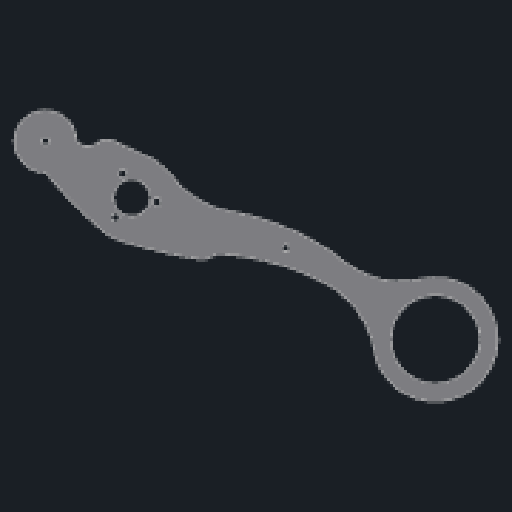
# Autodesk Inventor part: LowerLeg
Saved by Autodesk Inventor 2025.2 (Build 292293000, 293)
## iProperties
Created: 2020-05-17
Part Number: LowerLeg
Material: Generic
Document SubType Name: Sheet Metal
Designer: valer
Density: 1 g/cm^3
Sheet Metal Rule: Default
Appearance: Default
Author: valer
Autodesk Inventor part; units mm, degrees
ref_plane "YZ Plane" through (0, 0, 0) normal (1, 0, 0) x (0, 1, 0)
ref_plane "XZ Plane" through (0, 0, 0) normal (0, 1, 0) x (-1, 0, 0)
ref_plane "XY Plane" through (0, 0, 0) normal (0, 0, 1) x (1, 0, 0)
sketch "Base" plane through (0, 0, 0) normal (0, 0, 1) x (1, 0, 0)
  circle A0 centre (0, 0) radius 25.4
  arc A1 (296.4611, -175.8738) -> (140.4514, -91.7589) centre (131.6761, -294.7694) ccw
  arc A2 (110.2711, -36.5273) -> (55.3611, 0.3584) centre (-26.1088, -180.2356) ccw
  arc A3 (110.2711, -36.5273) -> (151.7939, -57.2356) centre (164.9104, 21.0482) ccw
  arc A4 (244.1, -98.1325) -> (151.7939, -57.2356) centre (118.2154, -257.642) ccw
  arc A5 (244.1, -98.1325) -> (322.9398, -136.302) centre (369.9847, 61.3771) ccw
  arc A6 (339.7063, -172.5127) -> (322.9398, -136.302) centre (317.0592, -161.0119) ccw
  arc A7 (296.4611, -175.8738) -> (339.7063, -172.5127) centre (317.0592, -161.0119) ccw
  line L0 (128.6011, -96.3262) -> (140.4514, -91.7589)
  line L1 (0, 0) -> (317.0592, -161.0119) construction
  circle A8 centre (317.0592, -161.0119) radius 25.4 construction
  arc A9 (0, -25.4) -> (128.6011, -96.3262) centre (153.166, 100.265) ccw
  line L2 (0, 0) -> (0, -25.4) construction
  arc A10 (55.3611, 0.3584) -> (42.3326, -1.2004) centre (50.1387, -11.2181) ccw
  arc A11 (25.4, -0.0141) -> (42.3326, -1.2004) centre (34.5266, 8.8174) ccw
  line L3 (110.2711, -36.5273) -> (102.4101, -52.0068) construction
  line L4 (50.1387, -11.2181) -> (44.3883, -22.5417) construction
  line L5 (140.4514, -91.7589) -> (148.7008, -75.5146) construction
  line L6 (244.1, -98.1325) -> (233.6726, -118.6658) construction
  line L7 (339.7063, -172.5127) -> (317.0592, -161.0119) construction
  dimension "d101" = 50.8
  dimension "d98" = 355.6
  dimension "d99" = 203.2
  dimension "d100" = 79.375
  dimension "d102" = 198.12
  dimension "d103" = 50.8
  dimension "d104" = 12.7
  dimension "d105" = 203.2
  dimension "d106" = 48
  dimension "d107" = 12.7
  dimension "d108" = 12.7
  dimension "d109" = 23.495
  dimension "d111" = 158.75
  dimension "d112" = 222.25
  dimension "d113" = 49.784
  dimension "d114" = 65.0748
  dimension "d115" = 51.9176
  dimension "d116" = 95.3008
  dimension "d117" = 93.5228
  measures "d98" distance of L1.start L1.end
  measures "d99" radius of A4
  measures "d100" radius of A3
  measures "d102" radius of A2
  measures "d103" diameter of A0
  measures "d104" radius of A10
  measures "d105" radius of A5
  measures "d106" angle of L1 L0
  measures "d107" distance of L0.start L0.end
  measures "d108" distance from line of L1 L4.start
  measures "d109" distance from line of L1 A11.centre
  measures "d111" distance from line of L1 A9.centre
  measures "d112" distance from line of L1 A5.centre
  measures "d113" distance from line of point (0, 0) L4
  measures "d114" distance from line of L4.end L3
  measures "d115" distance between parallel lines of L5 L3
  measures "d116" distance between parallel lines of L6 L5
  measures "d117" distance from line of A6.centre L6
extrude "Plate1" add sketch "Base" along normal blind 5
sketch "MountHoles" plane through (0, 0, 5) normal (0, 0, 1) x (1, 0, 0)
  arc A0 (296.4611, -175.8738) -> (322.9398, -136.302) centre (317.0592, -161.0119) ccw projected
  circle A1 centre (317.0592, -161.0119) radius 3.175
  circle A2 centre (0, 0) radius 3.175
  circle A3 centre (0, 0) radius 15.875 construction
  circle A4 centre (0, 15.875) radius 3.175
  line L0 (0, 15.875) -> (0, 0) construction
  circle A5 centre (-13.7482, 7.9375) radius 3.175
  circle A6 centre (-13.7482, -7.9375) radius 3.175
  circle A7 centre (0, -15.875) radius 3.175
  circle A8 centre (13.7482, -7.9375) radius 3.175
  circle A9 centre (13.7482, 7.9375) radius 3.175
  point P0 (278.6053, -195.7416)
  point P1 (14.9365, 6.9557)
  dimension "d40" = 31.75
  dimension "d38" = 6.35
  dimension "d39" = 6.35
  dimension "d43" = 360
  constraints: 8 centre point, 3 coincident, 2 end point, 1 equal radius, 1 vertical, 1 vertical alignment, 15 other
  measures "d38" diameter of A1
  measures "d39" diameter of A2
hole "MountHolesFeature" at (0, 0, 5) direction (0, 0, -1) diameter 6.35 end through all
fillet "SmallFilletsFeature" radius 8 2 edges at (140.4514, -91.7589, 2.5) (128.6011, -96.3262, 2.5)
sketch "WheelMountHole" plane through (0, 0, 5) normal (0, 0, 1) x (1, 0, 0)
  arc A0 (296.4611, -175.8738) -> (322.9398, -136.302) centre (317.0592, -161.0119) ccw projected
  circle A1 centre (317.0592, -161.0119) radius 6.35
  point P0 (0, 0)
  point P1 (278.6053, -195.7416)
  dimension "d83" = 12.7
  constraints: 1 centre point, 1 coincident
  measures "d83" diameter of A1
hole "WheelMountHoleFeature" at (317.0592, -161.0119, 5) direction (0, 0, -1) diameter 24.5 end through all
sketch "PistonMountHole" plane through (0, 0, 0) normal (0, 0, -1) x (-1, 0, 0)
  circle A0 centre (-195.6083, -86.6143) radius 3
  arc A1 (-151.7939, -57.2356) -> (-244.1, -98.1325) centre (-118.2154, -257.642) ccw projected
  line L0 (-206.4619, -74.6043) -> (-184.7548, -98.6243) construction
  arc A2 (-142.169, -91.8405) -> (-296.4611, -175.8738) centre (-131.6761, -294.7694) ccw projected
  point P0 (0, 0)
  dimension "d120" = 6
  dimension "d122" = 203.2
  constraints: 2 end point, 2 point on circle, 1 centre point, 1 coincident, 1 midpoint
  measures "d120" diameter of A0
  measures "d122" distance from line of point (0, 0) L0
extrude "PistonMountHoleFeature" cut sketch "PistonMountHole" against normal blind 5
sketch "MotorExtend" plane through (0, 0, 5) normal (0, 0, 1) x (1, 0, 0)
  circle A0 centre (70.2482, -45.9648) radius 36
  arc A1 (0, -25.4) -> (126.5447, -96.0583) centre (153.166, 100.265) ccw construction
  arc A2 (110.2711, -36.5273) -> (151.7939, -57.2356) centre (164.9104, 21.0482) ccw construction
  circle A3 centre (0, 0) radius 3.175
  line L0 (0, 0) -> (140.4963, -91.9296) construction
  arc A4 (142.169, -91.8405) -> (138.8789, -92.365) centre (141.7559, -99.8298) ccw
  arc A5 (0, -25.4) -> (46.966, -73.4228) centre (280.2614, 201.7164) ccw
  arc A6 (126.5447, -96.0583) -> (130.4966, -95.5956) centre (127.6196, -88.1308) ccw
  arc A7 (58.6335, -80.0397) -> (126.5447, -96.0583) centre (175.0163, 261.4034) ccw
  arc A8 (55.3611, 0.3584) -> (42.3326, -1.2004) centre (50.1387, -11.2181) ccw
  arc A9 (85.2601, -13.2441) -> (55.3611, 0.3584) centre (-2070.8473, -4712.7994) ccw
  arc A10 (110.2711, -36.5273) -> (55.3611, 0.3584) centre (-26.1088, -180.2356) ccw
  arc A11 (110.2711, -36.5273) -> (94.2542, -19.1374) centre (12.4591, -110.5454) ccw
  line L1 (0, -25.4) -> (55.3611, 0.3584)
  line L2 (110.2711, -36.5273) -> (126.5447, -96.0583)
  point P0 (70.2482, -45.9648)
  dimension "d128" = 72
  measures "d128" diameter of A0
sheet face with bend "MotorExtendFeature" sketch "MotorExtend" thickness 5 toward (0, 0, -1) bend radius 5 relief straight relief width 5 relief depth 2.5 contours A0 A10 | A11 A10 A0 | A0 A10 A9 | A10 L2 A7 A0 | A0 A10 | A0 A5 L1 A10
bend "Bend1"
sketch "MotorCut" plane through (0, 0, 5) normal (0, 0, 1) x (1, 0, 0)
  circle A0 centre (70.2482, -45.9648) radius 36 projected
  circle A1 centre (70.2482, -45.9648) radius 15
  point P0 (0, 0)
  dimension "d134" = 30
  constraints: 1 centre point, 1 coincident
  measures "d134" diameter of A1
extrude "MotorCutFeature" cut sketch "MotorCut" against normal blind 5 contours A1
sketch "MotorMountHoles" plane through (0, 0, 5) normal (0, 0, 1) x (1, 0, 0)
  circle A0 centre (56.943, -61.9327) radius 3.5 projected
  circle A1 centre (63.0721, -26.4582) radius 3.5 projected
  circle A2 centre (90.7293, -49.5034) radius 3.5 projected
  point P0 (0, 0)
extrude "MotorMountHolesFeature" cut sketch "MotorMountHoles" against normal blind 5
sketch "HubCoverExtend" plane through (0, 0, 5) normal (0, 0, 1) x (1, 0, 0)
  circle A0 centre (317.0592, -161.0119) radius 12.25
  circle A1 centre (317.0592, -161.0119) radius 50.8
  arc A2 (244.1, -98.1325) -> (322.9398, -136.302) centre (369.9847, 61.3771) ccw
  arc A3 (296.4611, -175.8738) -> (142.169, -91.8405) centre (131.6761, -294.7694) ccw
  arc A4 (244.1, -98.1325) -> (305.2545, -111.6025) centre (288.573, -41.7804) ccw
  arc A5 (266.9914, -169.606) -> (228.8665, -116.3198) centre (192.9202, -182.3202) ccw
  point P0 (0, 0)
  point P1 (283.7795, -122.6308)
  point P2 (268.8853, -144.8899)
  dimension "d139" = 101.6
  measures "d139" diameter of A1
sheet face with bend "HubCoverExtendFeature" sketch "HubCoverExtend" thickness 5 toward (0, 0, -1) bend radius 5 relief straight relief width 5 relief depth 2.5
bend "Bend2"
sketch "HubPressFitHole" plane through (0, 0, 5) normal (0, 0, 1) x (1, 0, 0)
  circle A0 centre (317.0592, -161.0119) radius 12.25 projected
  circle A1 centre (317.0592, -161.0119) radius 35.9873
  point P0 (0, 0)
  dimension "d145" = 71.9746
  constraints: 1 centre point, 1 coincident
  measures "d145" diameter of A1
extrude "HubPressFitHoleFeature" cut sketch "HubPressFitHole" against normal blind 5 contours A0 | A1
equation "\"d66\" = Thickness"
equation "\"d89\" = Thickness"
equation "\"d37\" = Thickness"
equation "\"BendRadius\" = Thickness"
equation "\"BendReliefWidth\" = Thickness"
equation "\"BendReliefDepth\" = 0.5 * Thickness"
equation "\"TransitionRadius\" = BendRadius"
equation "\"JacobiRadiusSize\" = BendRadius"
equation "\"GapSize\" = Thickness"
equation "\"Thickness\" = 5"
body "Solid1"
